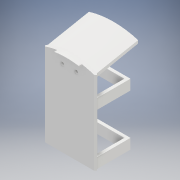
# Autodesk Inventor part: baseBateria
Saved by Autodesk Inventor 2017 (Build 210142000, 142)
## iProperties
Part Number: baseBateria
Material: Genérico
Document SubType Name: Modeling
Designer: Roberto
Density: 1 g/cm^3
Appearance: Valor por defecto
Author: Roberto
Autodesk Inventor part; units mm, degrees
ref_plane "YZ Plane" through (0, 0, 0) normal (1, 0, 0) x (0, 1, 0)
ref_plane "XZ Plane" through (0, 0, 0) normal (0, 1, 0) x (-1, 0, 0)
sketch "Boceto1" plane through (0, 0, 0) normal (0, 1, 0) x (-1, 0, 0)
  line L0 (4.8, 0) -> (4.8, 8.105632)
  line L1 (0, 0) -> (0, 8.105632)
  arc A0 (4.8, 8.105632) -> (0, 8.105632) centre (2.4, 1) ccw
  line L2 (0, 0) -> (4.8, 0)
  line L3 (4.8, 0) -> (4.5, 0)
  line L4 (4.5, 0) -> (4.5, 1)
  line L5 (4.5, 1) -> (4.8, 1)
  line L6 (4.8, 5) -> (4.5, 5)
  line L7 (4.5, 5) -> (4.5, 6)
  line L8 (4.5, 6) -> (4.8, 6)
  line L9 (0.3, 0) -> (0.3, 1)
  line L10 (0.3, 1) -> (0, 1)
  line L11 (0, 5) -> (0.3, 5)
  line L12 (0.3, 5) -> (0.3, 6)
  line L13 (0.3, 6) -> (0, 6)
  line L14 (0, 0) -> (1.4, 0)
  circle A1 centre (3.075, 7.5) radius 0.15
  circle A2 centre (1.725, 7.5) radius 0.15
  line L15 (2.55, 8.1985) -> (2.55, 0)
  line L16 (2.25, 8.1985) -> (2.25, 0)
  line L17 (0.9, 8.04847) -> (0.9, 0)
  line L18 (1.2, 8.103378) -> (1.2, 0)
  line L19 (3.9, 8.04847) -> (3.9, 0)
  line L20 (3.6, 8.103378) -> (3.6, 0)
  arc A3 (4.8, 7.805632) -> (0, 7.805632) centre (2.4, 0.7) ccw
  constraints: 40 end point, 11 point on line, 10 point on circle, 4 centre point, 12 other
extrude "Extrusión1" add sketch "Boceto1" along normal blind 0.3
sketch "Boceto2" plane through (0, 0.3, 0) normal (0, 1, 0) x (1, 0, 0)
  line L0 (-4.8, 0) -> (-4.8, -8.105632)
  line L1 (0, 0) -> (0, -8.105632)
  arc A0 (-4.8, -8.105632) -> (0, -8.105632) centre (-2.4, -1) ccw
  line L2 (0, 0) -> (-4.8, 0)
  line L3 (-4.8, 0) -> (-4.5, 0)
  line L4 (-4.5, 0) -> (-4.5, -1)
  line L5 (-4.5, -1) -> (-4.8, -1)
  line L6 (-4.8, -5) -> (-4.5, -5)
  line L7 (-4.5, -5) -> (-4.5, -6)
  line L8 (-4.5, -6) -> (-4.8, -6)
  line L9 (-0.3, 0) -> (-0.3, -1)
  line L10 (-0.3, -1) -> (0, -1)
  line L11 (0, -5) -> (-0.3, -5)
  line L12 (-0.3, -5) -> (-0.3, -6)
  line L13 (-0.3, -6) -> (0, -6)
  line L14 (0, 0) -> (-1.4, 0)
  circle A1 centre (-3.075, -7.5) radius 0.15
  circle A2 centre (-1.725, -7.5) radius 0.15
  line L15 (-2.55, -8.1985) -> (-2.55, 0)
  line L16 (-2.25, -8.1985) -> (-2.25, 0)
  line L17 (-0.9, -8.04847) -> (-0.9, 0)
  line L18 (-1.2, -8.103378) -> (-1.2, 0)
  line L19 (-3.9, -8.04847) -> (-3.9, 0)
  line L20 (-3.6, -8.103378) -> (-3.6, 0)
  arc A3 (-4.8, -7.805632) -> (0, -7.805632) centre (-2.4, -0.7) ccw
  point P0 (0, 0)
  constraints: 40 end point, 11 point on line, 10 point on circle, 4 centre point, 12 other
extrude "Extrusión2" add sketch "Boceto2" along normal blind 0.3 contours L2 L20 A3 L19 | L2 L16 A3 L15 | L2 L17 A3 L18
sketch "Boceto3" plane through (0, 0.3, 0) normal (0, 1, 0) x (1, 0, 0)
  line L0 (-4.8, 0) -> (-4.8, -8.105632)
  line L1 (0, 0) -> (0, -8.105632)
  arc A0 (-4.8, -8.105632) -> (0, -8.105632) centre (-2.4, -1) ccw
  line L2 (0, 0) -> (-4.8, 0)
  line L3 (-4.8, 0) -> (-4.5, 0)
  line L4 (-4.5, 0) -> (-4.5, -1)
  line L5 (-4.5, -1) -> (-4.8, -1)
  line L6 (-4.8, -5) -> (-4.5, -5)
  line L7 (-4.5, -5) -> (-4.5, -6)
  line L8 (-4.5, -6) -> (-4.8, -6)
  line L9 (-0.3, 0) -> (-0.3, -1)
  line L10 (-0.3, -1) -> (0, -1)
  line L11 (0, -5) -> (-0.3, -5)
  line L12 (-0.3, -5) -> (-0.3, -6)
  line L13 (-0.3, -6) -> (0, -6)
  line L14 (0, 0) -> (-1.4, 0)
  circle A1 centre (-3.075, -7.5) radius 0.15
  circle A2 centre (-1.725, -7.5) radius 0.15
  line L15 (-2.55, -8.1985) -> (-2.55, 0)
  line L16 (-2.25, -8.1985) -> (-2.25, 0)
  line L17 (-0.9, -8.04847) -> (-0.9, 0)
  line L18 (-1.2, -8.103378) -> (-1.2, 0)
  line L19 (-3.9, -8.04847) -> (-3.9, 0)
  line L20 (-3.6, -8.103378) -> (-3.6, 0)
  arc A3 (-4.8, -7.805632) -> (0, -7.805632) centre (-2.4, -0.7) ccw
  constraints: 40 end point, 11 point on line, 10 point on circle, 4 centre point, 12 other
extrude "Extrusión3" add sketch "Boceto3" along normal blind 3.25 contours L2 L4 L5 L0 | L6 L7 L8 L0 | L13 L12 L11 L1 | L2 L1 L10 L9
sketch "Boceto4" plane through (-4.5, 0.3, 6) normal (1, 0, 0) x (0, 0, -1)
  line L0 (1, 0) -> (0, 0) projected
  line L1 (1, 0) -> (1, 3.25) projected
  line L2 (0, 3.25) -> (1, 3.25) projected
  line L3 (0, 0) -> (0, 3.25) projected
  line L4 (6, 0) -> (5, 0) projected
  line L5 (6, 0) -> (6, 3.25) projected
  line L6 (5, 3.25) -> (6, 3.25) projected
  line L7 (5, 0) -> (5, 3.25) projected
  line L8 (0, 3.25) -> (0, 2.95)
  line L9 (0, 0) -> (0, 3.25) projected
  line L10 (0, 3.25) -> (1, 3.25) projected
  line L11 (1, 3.25) -> (1, 2.95)
  line L12 (1, 0) -> (1, 3.25) projected
  line L13 (1, 2.95) -> (0, 2.95)
  line L14 (1, 3.25) -> (0, 3.25)
  line L15 (5, 3.25) -> (5, 2.95)
  line L16 (6, 3.25) -> (6, 2.95)
  line L17 (6, 2.95) -> (5, 2.95)
  line L18 (6, 3.25) -> (5, 3.25)
  point P0 (6, -0.3)
  dimension "d6" = 0.3
  dimension "d7" = 0.3
  dimension "d8" = 0.3
  constraints: 16 end point, 2 point on line, 1 collinear
  measures "d6" distance of L2.start L8.end
  measures "d7" distance of L1.end L11.end
  measures "d8" distance of L15.start L15.end
extrude "Extrusión4" add sketch "Boceto4" along normal blind 4.2 contours L13 L3 L2 L1 | L17 L7 L6 L5
ref_plane "Plano de trabajo1" through (-2.4, 0, 8.105632) normal (1, 0, 0) x (0, 0, -1)
sketch "Boceto7" plane through (0, 0, 0) normal (0, 0, -1) x (-1, 0, 0)
  line L0 (0, 0) -> (4.8, 0) projected
  line L1 (3.9, 0.3) -> (4.5, 0.3) projected
  line L2 (4.925, 0.15) -> (4.8, 0.3)
  line L3 (4.925, 0.15) -> (4.8, 0)
  line L4 (4.8, 0.3) -> (4.8, 3.55) projected
  line L5 (4.8, 0.3) -> (0, 0.3)
  line L6 (-0.125, 0.15) -> (0, 0.3)
  line L7 (-0.125, 0.15) -> (0, 0)
  line L8 (4.8, 0) -> (0, 0) projected
  line L9 (0, 0) -> (4.8, 0)
  constraints: 12 end point, 1 collinear, 1 horizontal
extrude "Extrusión5" add sketch "Boceto7" against normal blind 9.2
sketch "Boceto8" plane through (0, 0.3, 0) normal (0, 1, 0) x (1, 0, 0)
  line L0 (-4.8, 0) -> (-4.8, -8.105632)
  line L1 (0, 0) -> (0, -8.105632)
  arc A0 (-4.8, -8.105632) -> (0, -8.105632) centre (-2.4, -1) ccw
  line L2 (0, 0) -> (-4.8, 0)
  line L3 (-4.8, 0) -> (-4.5, 0)
  line L4 (-4.5, 0) -> (-4.5, -1)
  line L5 (-4.5, -1) -> (-4.8, -1)
  line L6 (-4.8, -5) -> (-4.5, -5)
  line L7 (-4.5, -5) -> (-4.5, -6)
  line L8 (-4.5, -6) -> (-4.8, -6)
  line L9 (-0.3, 0) -> (-0.3, -1)
  line L10 (-0.3, -1) -> (0, -1)
  line L11 (0, -5) -> (-0.3, -5)
  line L12 (-0.3, -5) -> (-0.3, -6)
  line L13 (-0.3, -6) -> (0, -6)
  line L14 (0, 0) -> (-1.4, 0)
  circle A1 centre (-3.075, -7.5) radius 0.15
  circle A2 centre (-1.725, -7.5) radius 0.15
  line L15 (-2.55, -8.1985) -> (-2.55, 0)
  line L16 (-2.25, -8.1985) -> (-2.25, 0)
  line L17 (-0.9, -8.04847) -> (-0.9, 0)
  line L18 (-1.2, -8.103378) -> (-1.2, 0)
  line L19 (-3.9, -8.04847) -> (-3.9, 0)
  line L20 (-3.6, -8.103378) -> (-3.6, 0)
  arc A3 (-4.8, -7.805632) -> (0, -7.805632) centre (-2.4, -0.7) ccw
  arc A4 (-4.8, -8.105632) -> (0, -8.105632) centre (-2.4, -1) ccw
  arc A5 (-5.931931, -7.616303) -> (1.068069, -7.65) centre (-2.4, -1) ccw
  line L21 (1.068069, -7.65) -> (1.068069, -11.446535)
  line L22 (1.068069, -11.446535) -> (-5.931931, -11.446535)
  line L23 (-5.931931, -11.446535) -> (-5.931931, -7.616303)
  point P0 (0, 0)
  point P1 (0, 0)
  dimension "d20" = 7
  constraints: 46 end point, 14 point on circle, 11 point on line, 6 centre point, 2 perpendicular, 1 coincident, 1 vertical, 12 other
  measures "d20" distance of L21.end L22.end
extrude "Extrusión6" cut sketch "Boceto8" against normal blind 9.2 contours A0 A5 L21 L22 L23
sketch "Boceto10" plane through (-2.4, 0, 8.105632) normal (1, 0, 0) x (0, 0, -1)
  line L0 (-0.394368, 0.3) -> (-0.088768, 0.3)
  line L1 (-0.866282, 4.3) -> (-0.088768, 0.3)
  line L2 (-1.137405, 4.3) -> (-0.394368, 0.3)
  arc A0 (2.945532, 14.9949) -> (-1.390306, 6.995896) centre (6.669532, 7.8017) ccw
  arc A1 (2.834168, 15.209576) -> (-1.627568, 6.9387) centre (6.669532, 7.8017) ccw
  line L3 (-0.394368, 0.3) -> (14.605632, 0.3)
  line L4 (7.105632, 16.0708) -> (7.105632, 16.312794)
  arc A2 (7.105632, 16.0708) -> (2.878317, 14.959702) centre (7.380132, 6.4292) ccw
  arc A3 (7.105632, 16.312794) -> (2.834168, 15.209576) centre (7.380132, 6.4292) ccw
  line L5 (-0.394368, 0.3) -> (-0.088768, 0.3)
  line L6 (-0.088768, 0.3) -> (-0.866282, 4.3)
  line L7 (-1.137405, 4.3) -> (-0.394368, 0.3)
  line L8 (-1.627568, 6.9387) -> (-1.390306, 6.995896)
  line L9 (7.105632, 16.312794) -> (7.105632, 16.0708)
  line L10 (-0.394368, 0) -> (-0.394368, 0.3)
  line L11 (-1.137405, 4.3) -> (-0.866282, 4.3)
  point P0 (-0.394368, 0.3)
  dimension "d24" = 15
  constraints: 22 end point, 11 point on circle, 4 centre point, 3 collinear, 2 coincident, 2 horizontal, 1 perpendicular, 1 vertical
  measures "d24" distance of L3.start L3.end
revolve "Revolución2" add sketch "Boceto10" angle 39 mid plane about axis through (-2.4, 16.0708, 1) along (0, 1, 0) contours L2 L11 L1 L0
sketch "Boceto11" plane through (0, 0.3, 7.782285) normal (0, -1, 0) x (1, 0, 0)
  line L0 (0, -7.782285) -> (0, 0.323346)
  arc A0 (0.103551, 0.287526) -> (0, 0.323346) centre (-2.4, -6.782285) ccw
  line L1 (0.103551, 0.287526) -> (0.00154, -0.000545)
  line L2 (0, 0) -> (0, -1.782285)
  line L3 (0, 0) -> (0, 0.323346)
  line L4 (0, 0) -> (0, 0.788646)
  line L5 (0, 0.788646) -> (0, 1.874825)
  line L6 (0, 1.874825) -> (1.415371, 1.874825)
  line L7 (1.415371, 1.874825) -> (1.415371, 0)
  line L8 (0, 0) -> (1.415371, 0)
  line L9 (-4.8, 0) -> (-4.8, 0.323346)
  line L10 (0, 0) -> (-4.8, 0)
  line L11 (-2.4, 0) -> (-2.4, 5.52378)
  line L12 (-4.8, 0) -> (-4.8, 0.788646)
  line L13 (-4.8, 0.788646) -> (-4.8, 1.874825)
  line L14 (-4.8, 1.874825) -> (-6.215371, 1.874825)
  line L15 (-6.215371, 1.874825) -> (-6.215371, 0)
  line L16 (-4.8, 0) -> (-6.215371, 0)
  constraints: 26 end point, 4 perpendicular, 4 symmetric about line, 2 point on line, 2 vertical, 1 collinear, 1 midpoint
extrude "Extrusión7" cut sketch "Boceto11" against normal blind 9.2
sketch "Boceto12" plane through (0, 0, 0) normal (0, -1, 0) x (1, 0, 0)
  line L0 (0, 0) -> (0, 8.105632)
  line L1 (-4.8, 0) -> (-4.8, 8.105632)
  arc A0 (0, 8.105632) -> (-4.8, 8.105632) centre (-2.4, 1) ccw
  line L2 (-4.8, 0) -> (0, 0)
  line L3 (0, 0) -> (-0.3, 0)
  line L4 (-0.3, 0) -> (-0.3, 1)
  line L5 (-0.3, 1) -> (0, 1)
  line L6 (0, 5) -> (-0.3, 5)
  line L7 (-0.3, 5) -> (-0.3, 6)
  line L8 (-0.3, 6) -> (0, 6)
  line L9 (-4.5, 0) -> (-4.5, 1)
  line L10 (-4.5, 1) -> (-4.8, 1)
  line L11 (-4.8, 5) -> (-4.5, 5)
  line L12 (-4.5, 5) -> (-4.5, 6)
  line L13 (-4.5, 6) -> (-4.8, 6)
  line L14 (-4.8, 0) -> (-3.4, 0)
  circle A1 centre (-1.725, 7.5) radius 0.15
  circle A2 centre (-3.075, 7.5) radius 0.15
  line L15 (-2.25, 8.1985) -> (-2.25, 0)
  line L16 (-2.55, 8.1985) -> (-2.55, 0)
  line L17 (-3.9, 8.04847) -> (-3.9, 0)
  line L18 (-3.6, 8.103378) -> (-3.6, 0)
  line L19 (-0.9, 8.04847) -> (-0.9, 0)
  line L20 (-1.2, 8.103378) -> (-1.2, 0)
  arc A3 (0, 7.805632) -> (-4.8, 7.805632) centre (-2.4, 0.7) ccw
  point P0 (-4.8, 0)
  constraints: 40 end point, 11 point on line, 10 point on circle, 4 centre point, 12 other
extrude "Extrusión8" cut sketch "Boceto12" against normal blind 10 contours A1 | A2
sketch "Boceto14" plane through (0, 0, 0) normal (0, -1, 0) x (1, 0, 0)
  arc A0 (0, 8.105632) -> (-4.8, 8.105632) centre (-2.4, 1) ccw
  arc A1 (-1.2, 8.15) -> (-3.6, 8.15) centre (-2.4, 1) ccw
  line L0 (-1.2, 8.403378) -> (-1.2, 8.15)
  line L1 (-3.6, 8.403378) -> (-3.6, 8.15)
  arc A2 (-1.2, 8.403378) -> (-3.6, 8.403378) centre (-2.4, 1) ccw
  point P0 (0, 0)
  dimension "d34" = 0.25
  constraints: 6 point on circle, 4 end point, 2 centre point, 1 concentric
  measures "d34" radial gap between concentric circles of A0 A1
extrude "Extrusión10" add sketch "Boceto14" along normal blind 0.3
chamfer "Chaflán1" distance 0.2 angle 45 1 edges at (-2.4, -0.3, 8.25)
